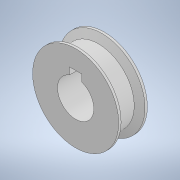
# Autodesk Inventor part: Pulley
Saved by Autodesk Inventor 2022 (Build 260153000, 153)
## iProperties
Created: 2022-08-17
Part Number: Pulley
Material: Generic
Document SubType Name: Modeling
Designer: Nick
Density: 1 g/cm^3
Appearance: Default
Mass: 9.79549 g
Surface Area: 47.4538 cm^2
Volume: 9.79549 cm^3
Author: Nick
Autodesk Inventor part; units mm, degrees
ref_plane "YZ Plane" through (0, 0, 0) normal (1, 0, 0) x (0, 1, 0)
ref_plane "XZ Plane" through (0, 0, 0) normal (0, 1, 0) x (-1, 0, 0)
ref_plane "XY Plane" through (0, 0, 0) normal (0, 0, 1) x (1, 0, 0)
sketch "Sketch4" plane through (0, 0, 0) normal (0, 0, 1) x (1, 0, 0)
  circle A0 centre (0, 0) radius 7.5
  circle A1 centre (0, 0) radius 15
  line L0 (-2.5, 10) -> (2.5, 10)
  line L1 (2.5, 10) -> (2.5, 5)
  line L2 (2.5, 5) -> (-2.5, 5)
  line L3 (-2.5, 5) -> (-2.5, 10)
  point P0 (0, 7.5)
  point P1 (2.5, 7.5)
  point P2 (0, 5)
  point P3 (2.5, 7.0711)
  point P4 (-2.5, 7.0711)
  dimension "d17" = 15
  dimension "d18" = 5
  dimension "d19" = 5
  dimension "d20" = 30
  constraints: 8 end point, 2 coincident, 2 midpoint, 2 parallel, 2 vertical alignment, 1 centre point, 1 horizontal, 1 horizontal alignment, 1 perpendicular, 3 other
  measures "d18" distance of L1.end L2.end
  measures "d19" distance of L0.end L1.end
  measures "d20" diameter of A1
extrude "Extrusion3" add sketch "Sketch4" along normal blind 12
sketch "Sketch5" plane through (0, 0, 0) normal (1, 0, 0) x (0, 1, 0)
  line L0 (15, 12) -> (-15, 12) projected
  line L1 (15, 0) -> (-15, 0) projected
  line L2 (15, 12) -> (-15, 12) projected
  line L3 (15, 12) -> (18, 12)
  line L4 (18, 12) -> (18, 11)
  line L5 (18, 11) -> (15, 9.5)
  line L6 (15, 9.5) -> (15, 2.5)
  line L7 (15, 2.5) -> (18, 1)
  line L8 (18, 1) -> (18, 0)
  line L9 (15, 0) -> (-15, 0) projected
  line L10 (18, 0) -> (15, 0)
  line L11 (15, 0) -> (15, 12) projected
  line L12 (0, -2.4) -> (0, 14.4) projected
  point P0 (0, 0)
  point P1 (15, 6)
  point P2 (15, 6)
  dimension "d23" = 7
  dimension "d24" = 3
  dimension "d25" = 1
  dimension "d26" = 1
  constraints: 14 end point, 3 point on line, 2 collinear, 2 midpoint, 1 coincident, 1 parallel, 1 perpendicular
  measures "d23" distance of L5.end L6.end
  measures "d24" distance of L0.start L3.end
  measures "d25" distance of L7.end L8.end
  measures "d26" distance of L3.end L4.end
revolve "Revolution1" add sketch "Sketch5" angle 360 about axis through (0, 0, -10) along (0, 0, 1) contours L3 L4 L5 L11 | L7 L8 L10 L11
thicken "Thicken1" operation add thickness 0.1 both sides no extend neighbours yes toward (-0.4087164, 0.9126614, 0) faces at (-3.0654, 6.845, 8) (2.5, 9.0237, 4) (-0.8333, 10, 4) (-2.5, 8.0474, 8)
body "Solid2"
